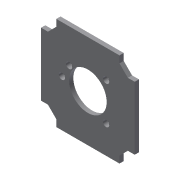
# Autodesk Inventor part: 20_Cube_insert_Sample_holder
Saved by Autodesk Inventor 2019 (Build 230136000, 136)
## iProperties
Created: 2019-08-07
Part Number: 20_Cube_insert_Sample_holder
Material: Generic
Document SubType Name: Modeling
Designer: marsikovabarbora
Density: 1 g/cm^3
Appearance: Default
Author: marsikovabarbora
Autodesk Inventor part; units mm, degrees
ref_plane "YZ Plane" through (0, 0, 0) normal (1, 0, 0) x (0, 1, 0)
ref_plane "Work Plane1" through (-29.1, -14.5, 2.4) normal (0, 0, -1) x (0, 1, 0)
ref_plane "Work Plane2" through (-13.8999, -10.5497, 2.25) normal (0, 0, -1) x (0, 1, 0)
sketch "Sketch1" plane through (0, 0, 0) normal (0, 0, 1) x (1, 0, 0)
  line L0 (-34.86, 0) -> (34.86, 0) construction
  line L1 (0, -34.86) -> (0, 34.86) construction
  line L2 (0, 0) -> (11.1575, 11.1575) construction
  line L3 (0, 0) -> (15.7791, 0) construction
  line L4 (0, 24.9) -> (16.8009, 24.9)
  line L5 (16.8009, 24.9) -> (16.8009, 21.2415)
  line L6 (16.8009, 21.2415) -> (19.0212, 19.0212)
  line L7 (24.9, 0) -> (24.9, 16.8009)
  line L8 (24.9, 16.8009) -> (21.2415, 16.8009)
  line L9 (21.2415, 16.8009) -> (19.0212, 19.0212)
  line L10 (0, -24.9) -> (16.8009, -24.9)
  line L11 (16.8009, -24.9) -> (16.8009, -21.2415)
  line L12 (16.8009, -21.2415) -> (19.0212, -19.0212)
  line L13 (24.9, 0) -> (24.9, -16.8009)
  line L14 (24.9, -16.8009) -> (21.2415, -16.8009)
  line L15 (21.2415, -16.8009) -> (19.0212, -19.0212)
  line L16 (0, 24.9) -> (-16.8009, 24.9)
  line L17 (-16.8009, 24.9) -> (-16.8009, 21.2415)
  line L18 (-16.8009, 21.2415) -> (-19.0212, 19.0212)
  line L19 (-24.9, 16.8009) -> (-21.2415, 16.8009)
  line L20 (-21.2415, 16.8009) -> (-19.0212, 19.0212)
  line L21 (0, -24.9) -> (-16.8009, -24.9)
  line L22 (-16.8009, -24.9) -> (-16.8009, -21.2415)
  line L23 (-16.8009, -21.2415) -> (-19.0212, -19.0212)
  line L24 (-21.2415, -16.8009) -> (-19.0212, -19.0212)
  line L25 (-24.9, -16.8009) -> (-21.2415, -16.8009)
  line L26 (-24.9, 0) -> (-24.9, -16.8009)
  line L27 (-24.9, 0) -> (-24.9, 16.8009)
  circle A0 centre (0, 0) radius 10
  dimension "d0" = 45
  dimension "d2" = 24.9
  dimension "d3" = 3.14
  dimension "d4" = 26.9
  dimension "d5" = 20
  constraints: 52 end point, 20 symmetric about line, 2 horizontal, 2 perpendicular, 2 point on line, 1 centre point, 1 coincident, 1 equal length
  measures "d0" angle of L3 L2
  measures "d2" distance between parallel lines of L0 L4
  measures "d3" distance of L5.end L6.end
  measures "d4" distance from line of L2.start L6
  measures "d5" diameter of A0
extrude "Extrusion1" add sketch "Sketch1" along normal up to surface (2.25 mm away)
sketch "Sketch5" plane through (0, 0, 0) normal (0, 0, -1) x (-1, 0, 0)
  circle A0 centre (-9.7, 10) radius 1.4
  circle A1 centre (-9.7, -10) radius 1.4
  circle A2 centre (13.8, 0) radius 1.4
  circle A3 centre (-10, 6.9) radius 0.75
  circle A4 centre (10, 6.9) radius 1.25
  point P0 (0, 0)
  constraints: 5 centre point, 10 other
hole "Hole1" at (-13.8, 0, 0) at (9.7, -10, 0) at (-10, 6.9, 0) at (9.7, 10, 0) direction (0, 0, 1) diameter 3.3 depth 12 tip angle 118
body "Solid1"
